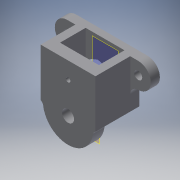
# Autodesk Inventor part: Bracket
Saved by Autodesk Inventor 2019 (Build 230136000, 136)
## iProperties
Created: 2021-03-26
Part Number: Bracket
Material: Generic
Document SubType Name: Modeling
Designer: Ian
Density: 1 g/cm^3
Appearance: Default
Author: Ian
Autodesk Inventor part; units mm, degrees
note: some values were not read from the file. Chosen so that the rebuilt part matches the saved one: arc direction of "Extrusion1".
ref_plane "Work Plane1" through (0, 0, 0.1) normal (0, 0, 1) x (1, 0, 0)
sketch "Sketch2" plane through (0, 0, 0.1) normal (0, 0, 1) x (1, 0, 0)
  arc A0 (-1.5411, 2.125) -> (1.5411, 2.125) centre (0, 0) ccw construction
  line L0 (-1.5411, 2.125) -> (1.5411, 2.125) construction
  circle A1 centre (0, 0) radius 8 construction
  line L1 (1.5, 2) -> (-1.5, 2) construction
  arc A2 (-1.5, 2) -> (1.5, 2) centre (0, 0) ccw construction
  circle A3 centre (0, 0) radius 11 projected
  circle A4 centre (-15.5, -15.5) radius 1.75 construction
  circle A5 centre (15.5, -15.5) radius 1.75 construction
  circle A6 centre (15.5, 15.5) radius 1.75 construction
  circle A7 centre (-15.5, 15.5) radius 1.75 construction
  line L2 (-21, 21) -> (21, 21) construction
  line L3 (-21, -21) -> (-21, 21) construction
  line L4 (21, -21) -> (-21, -21) construction
  line L5 (21, 21) -> (21, -21) construction
  line L6 (-11, 0) -> (-11, 21)
  line L7 (-11, 21) -> (11, 21)
  line L8 (11, 21) -> (11, 0)
  circle A8 centre (0, 0) radius 2.625
  dimension "d0" = 5.25
  constraints: 6 end point, 2 perpendicular, 2 point on circle, 2 point on line, 2 tangent, 1 centre point, 1 coincident
  measures "d0" diameter of A8
extrude "Extrusion1" add sketch "Sketch2" along normal blind 5
sketch "Sketch3" plane through (0, 0, 0.1) normal (0, 0, -1) x (-1, 0, 0)
  circle A0 centre (0, 13.698) radius 2.2 projected
  circle A1 centre (0, 13.698) radius 2
  point P0 (0, 0)
  dimension "d3" = 4
  constraints: 1 centre point, 1 coincident
  measures "d3" diameter of A1
extrude "Extrusion2" cut sketch "Sketch3" against normal blind 3 contours A1
sketch "Sketch4" plane through (0, 13.698, 3.1) normal (0, 0, -1) x (-1, 0, 0)
  circle A0 centre (0, 0) radius 1
  circle A1 centre (0, 0) radius 2 projected
  point P0 (0, -13.698)
  dimension "d6" = 2
  constraints: 1 centre point, 1 concentric
  measures "d6" diameter of A0
extrude "Extrusion3" cut sketch "Sketch4" against normal through all contours A0
sketch "Sketch5" plane through (0, 0, 0.1) normal (0, 0, -1) x (-1, 0, 0)
  circle A0 centre (0, 0) radius 8 construction
  line L0 (-8, 0) -> (-8, 21) construction
  line L1 (-11, 21) -> (11, 21) construction
  line L2 (8, 0) -> (8, 21) construction
  line L3 (-8.5, 0) -> (-8.5, 21) construction
  line L4 (8.5, 0) -> (8.5, 21) construction
  circle A1 centre (0, 0) radius 8.5 construction
  line L5 (-8.5, 0) -> (-12, 0)
  line L6 (-12, 0) -> (-12, 21)
  line L7 (-12, 21) -> (-8.5, 21)
  line L8 (-8.5, 21) -> (-8.5, 0)
  line L9 (8.5, 0) -> (12, 0)
  line L10 (12, 0) -> (12, 21)
  line L11 (12, 21) -> (8.5, 21)
  line L12 (8.5, 21) -> (8.5, 0)
  line L13 (11, 21) -> (-11, 21) projected
  dimension "d9" = 0.5
  dimension "d10" = 0.5
  dimension "d11" = 0.5
  dimension "d12" = 3.5
  dimension "d13" = 3.5
  constraints: 24 end point, 7 parallel, 3 point on line, 2 collinear, 2 horizontal, 2 perpendicular, 2 point on circle, 2 tangent, 1 centre point, 1 horizontal alignment, 1 vertical
  measures "d9" distance between parallel lines of L0 L3
  measures "d10" distance between parallel lines of L2 L4
  measures "d11" radial gap between concentric circles of A0 A1
  measures "d12" distance of L6.end L7.end
  measures "d13" distance of L10.end L11.end
ref_plane "Work Plane2" through (-11, -11, -12.1) normal (0, 0, 1) x (1, 0, 0)
extrude "Extrusion4" add sketch "Sketch5" along normal up to surface (12.2 mm away)
sketch "Sketch6" plane through (0, 0, 0.1) normal (0, 0, 1) x (1, 0, 0)
  line L0 (-11, 0) -> (-11, 21) projected
  line L1 (-11, 21) -> (-12, 21) projected
  line L2 (-12, 21) -> (-12, 0) projected
  line L3 (-12, 0) -> (-11, 0) projected
  line L4 (11, 21) -> (11, 0) projected
  line L5 (11, 0) -> (12, 0) projected
  line L6 (12, 0) -> (12, 21) projected
  line L7 (12, 21) -> (11, 21) projected
  point P0 (0, 0)
extrude "Extrusion5" add sketch "Sketch6" along normal up to surface (5 mm away)
fillet "Fillet1" radius 2 2 edges at (11, 0, 2.6) (-11, 0, 2.6)
sketch "Sketch7" plane through (12, 0, -12.1) normal (0, 0, -1) x (-1, 0, 0)
  circle A0 centre (12, 0) radius 11 projected
  line L0 (33, 21) -> (-9, 21) construction
  circle A1 centre (27.5, -15.5) radius 1.75 construction
  circle A2 centre (-3.5, -15.5) radius 1.75 construction
  circle A3 centre (-3.5, 15.5) radius 1.75 construction
  circle A4 centre (27.5, 15.5) radius 1.75 construction
  line L1 (33, 21) -> (-9, 21) construction
  line L2 (-9, 21) -> (-9, -21) construction
  line L3 (-9, -21) -> (33, -21) construction
  line L4 (33, -21) -> (33, 21) construction
  circle A5 centre (-3.5, 15.5) radius 1.75 projected
  arc A6 (-3.5, 21) -> (-3.5, 10) centre (-3.5, 15.5) ccw
  line L5 (0, 21) -> (0, 0) projected
  arc A7 (0, 6.5) -> (-3.5, 10) centre (-3.5, 6.5) ccw
  line L6 (24, 21) -> (0, 21) projected
  line L7 (-3.5, 21) -> (0, 21)
  arc A8 (1.1058, -1.5218) -> (0, 0) centre (-0.875, -1.7984) ccw projected
  arc A9 (24, 0) -> (22.8942, -1.5218) centre (24.875, -1.7984) ccw projected
  line L8 (24, 0) -> (24, 21) projected
  circle A10 centre (12, 0) radius 12
  line L9 (0, 0) -> (3.5, 0) projected
  line L10 (0, 6.5) -> (0, 0)
  line L11 (0, 21) -> (12, 21)
  line L12 (20.5, 21) -> (3.5, 21) projected
  line L13 (12, 21) -> (12, 14.698)
  circle A11 centre (12, 13.698) radius 1 projected
  line L14 (12, 12.698) -> (12, 12)
  arc A12 (12, 12) -> (0, 0) centre (12, 0) ccw
  arc A13 (12, 14.698) -> (12, 12.698) centre (12, 13.698) ccw
  point P0 (12, 0)
  point P1 (-3.125, 21)
  constraints: 10 end point, 10 point on circle, 4 centre point, 4 point on line, 4 tangent, 2 concentric, 2 vertical, 2 vertical alignment, 1 collinear, 1 midpoint, 1 perpendicular, 3 other
ref_plane "Work Plane3" through (-21, -21, -14.1) normal (0, 0, 1) x (1, 0, 0)
extrude "Extrusion6" add sketch "Sketch7" along normal up to surface (2 mm away) contours L5 L6 L13 A11 L14 A10 | A7 A6 L7 L5
mirror "Mirror1" about plane through (0, 14.698, -12.1) normal (-1, 0, 0) of "Extrusion6"
ref_plane "Work Plane4" through (0, 13.698, -11.1) normal (0, 0, -1) x (-1, 0, 0)
sketch "Sketch9" plane through (0, 13.698, -11.1) normal (0, 0, -1) x (-1, 0, 0)
  circle A0 centre (0, 0) radius 5.2 projected
  circle A1 centre (0, 0) radius 2
  line L0 (-8.5, 7.302) -> (8.5, 7.302) projected
  line L1 (8.5, 7.302) -> (8.5, -5.2275) projected
  arc A2 (8.5, -5.2275) -> (-8.5, -5.2275) centre (0, -13.698) ccw projected
  line L2 (-8.5, -5.2275) -> (-8.5, 7.302) projected
  circle A3 centre (0, 0) radius 1 projected
  arc A4 (8.5, -5.2275) -> (-8.5, -5.2275) centre (0, -13.698) ccw projected
  arc A5 (8.5, -5.2275) -> (0.9883, -1.7388) centre (0, -13.698) ccw
  arc A6 (-0.9883, -1.7388) -> (-8.5, -5.2275) centre (0, -13.698) ccw
  arc A7 (0.9883, -1.7388) -> (-0.9883, -1.7388) centre (0, 0) ccw
  line L3 (-12, 7.302) -> (-12, -7.198) projected
  arc A8 (-12, -7.198) -> (-15.5, -3.698) centre (-15.5, -7.198) ccw projected
  arc A9 (-15.5, 7.302) -> (-15.5, -3.698) centre (-15.5, 1.802) ccw projected
  line L4 (-12, 7.302) -> (-15.5, 7.302) projected
  point P0 (0, -13.698)
  dimension "d26" = 4
  constraints: 10 point on circle, 4 centre point, 1 coincident, 1 concentric
  measures "d26" diameter of A1
extrude "Extrusion8" add sketch "Sketch9" along normal up to surface (1 mm away) contours A0 A2 A1 | A0 A2 L2 L0 L1 | A1 A2 | A3 picked at (-3.5209, -0.8252) picked at (-0.5576, -1.4588)
sketch "Sketch10" plane through (12, 0, -12.1) normal (0, 0, 1) x (1, 0, 0)
  circle A0 centre (-12, 13.698) radius 1 projected
  circle A1 centre (-12, 13.698) radius 2
  point P0 (-12, 0)
  dimension "d29" = 4
  constraints: 1 centre point, 1 coincident
  measures "d29" diameter of A1
extrude "Extrusion9" cut sketch "Sketch10" against normal through all
sketch "Sketch11" plane through (-8.5, 0, -12.1) normal (0, 0, -1) x (-1, 0, 0)
  circle A0 centre (-8.5, 0) radius 11 construction
  arc A1 (-20.5, 0) -> (-20.5, 0) centre (-8.5, 0) ccw construction
  arc A2 (3.5, 0) -> (-20.5, 0) centre (-8.5, 0) ccw construction
  arc A3 (-9.4883, 11.9592) -> (-17, 8.4705) centre (-8.5, 0) ccw construction
  arc A4 (-11.5525, 11.6053) -> (-5.4475, 11.6053) centre (-8.5, 19) ccw
  circle A5 centre (-8.5, 13.698) radius 2 construction
  arc A6 (-9.4883, 11.9592) -> (-7.5117, 11.9592) centre (-8.5, 13.698) ccw
  arc A7 (-5.4475, 11.6053) -> (-7.5117, 11.9592) centre (-8.5, 0) ccw
  arc A8 (-9.4883, 11.9592) -> (-11.5525, 11.6053) centre (-8.5, 0) ccw
  point P0 (-8.5, 0)
  dimension "d32" = 8
  constraints: 10 point on circle, 4 centre point, 2 concentric, 2 tangent, 1 horizontal alignment, 1 other
  measures "d32" radius of A4
ref_plane "Work Plane5" through (-21, -21, -14.1) normal (0, 0, 1) x (1, 0, 0)
extrude "Extrusion10" add sketch "Sketch11" along normal up to surface (2 mm away)
sketch "Sketch12" plane through (-8.5, 0, -12.1) normal (0, 0, 1) x (1, 0, 0)
  arc A0 (7.5117, 11.9592) -> (9.4883, 11.9592) centre (8.5, 13.698) ccw projected
  arc A1 (7.5117, 11.9592) -> (5.4475, 11.6053) centre (8.5, 0) ccw projected
  arc A2 (5.4475, 11.6053) -> (11.5525, 11.6053) centre (8.5, 19) ccw projected
  arc A3 (11.5525, 11.6053) -> (9.4883, 11.9592) centre (8.5, 0) ccw projected
  point P0 (8.5, 0)
extrude "Extrusion11" add sketch "Sketch12" along normal up to surface (1 mm away)
sketch "Sketch13" plane through (12, 0, -12.1) normal (0, 0, 1) x (1, 0, 0)
  line L0 (0, 21) -> (0, 6.5) projected
  arc A0 (3.5, 10) -> (0, 6.5) centre (3.5, 6.5) ccw projected
  arc A1 (3.5, 10) -> (3.5, 21) centre (3.5, 15.5) ccw projected
  line L1 (0, 21) -> (3.5, 21) projected
  circle A2 centre (3.5, 15.5) radius 1.75 projected
  line L2 (-24, 6.5) -> (-24, 21) projected
  line L3 (-24, 21) -> (-27.5, 21) projected
  arc A3 (-27.5, 21) -> (-27.5, 10) centre (-27.5, 15.5) ccw projected
  arc A4 (-24, 6.5) -> (-27.5, 10) centre (-27.5, 6.5) ccw projected
  circle A5 centre (-27.5, 15.5) radius 1.75 projected
  point P0 (-12, 0)
extrude "Extrusion12" add sketch "Sketch13" along normal blind 2
body "Solid1"
